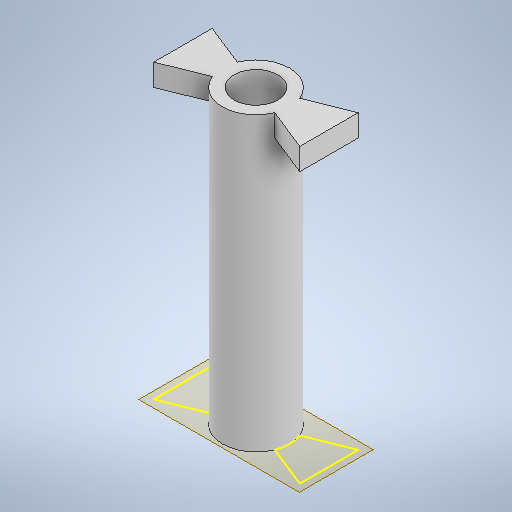
# Autodesk Inventor part: PruebaBuje
Saved by Autodesk Inventor 2025.2 (Build 292293000, 293)
## iProperties
Created: 2025-04-03
Part Number: PruebaBuje
Material: Genérico
Document SubType Name: Modeling
Designer: braug
Density: 1 g/cm^3
Appearance: Valor por defecto
Author: braug
## iProperties of the stored document PruebaBuje_3DPrint.ipt
Created: 2025-04-03
Part Number: PruebaBuje_3DPrint
Material: Genérico
Document SubType Name: Modeling
Designer: braug
Density: 1 g/cm^3
Appearance: Valor por defecto
Author: braug
Autodesk Inventor part; units mm, degrees
ref_plane "YZ Plane" through (0, 0, 0) normal (1, 0, 0) x (0, 1, 0)
ref_plane "XY Plane" through (0, 0, 0) normal (0, 0, 1) x (1, 0, 0)
sketch "Boceto1" plane through (0, 0, 0) normal (0, 1, 0) x (-1, 0, 0)
  circle A0 centre (0, 0) radius 1.5
  circle A1 centre (0, 0) radius 2.3
  dimension "d0" = 3
  dimension "d1" = 4.6
  constraints: 2 centre point, 2 coincident
  measures "d0" diameter of A0
  measures "d1" diameter of A1
extrude "Extrusión1" add sketch "Boceto1" along normal blind 20
sketch "Boceto2" plane through (0, 20, 0) normal (0, 1, 0) x (1, 0, 0)
  line L0 (5, 2) -> (5, -2)
  line L1 (-5, -2) -> (-5, 2)
  circle A0 centre (0, 0) radius 1.5 projected
  line L2 (-5, 2) -> (5, -2) construction
  line L3 (5, 2) -> (-5, -2) construction
  circle A1 centre (0, 0) radius 2.3 projected
  line L4 (-2.1355, 0.8542) -> (-5, 2)
  line L5 (-2.1355, -0.8542) -> (-5, -2)
  line L6 (2.1355, 0.8542) -> (5, 2)
  line L7 (5, -2) -> (2.1355, -0.8542)
  arc A2 (-2.1355, 0.8542) -> (-2.1355, -0.8542) centre (0, 0) ccw
  arc A3 (2.1355, -0.8542) -> (1.6097, 1.6429) centre (0, 0) ccw
  dimension "d5" = 4
  dimension "d8" = 10
  constraints: 16 end point, 8 point on circle, 4 point on line, 2 centre point, 2 collinear, 2 midpoint, 1 coincident, 1 parallel
  measures "d5" distance of L0.start L0.end
  measures "d8" distance between parallel lines of L1 L0
extrude "Extrusión2" add sketch "Boceto2" against normal blind 1.5 contours L0 L7 A1 L6 | L5 L1 L4 A1
sketch "Boceto3" plane through (0, 0, 0) normal (0, -1, 0) x (1, 0, 0)
  line L0 (-2.1355, 0.8542) -> (-5, 2) projected
  line L1 (-5, 2) -> (-5, -2) projected
  line L2 (-2.1355, 0.8542) -> (-5, 2) projected
  line L3 (-5, 2) -> (-5, -2) projected
  line L4 (-5, -2) -> (-2.1355, -0.8542) projected
  arc A0 (-2.1355, 0.8542) -> (-2.1355, -0.8542) centre (0, 0) ccw projected
  line L5 (2.1355, -0.8542) -> (5, -2) projected
  line L6 (5, -2) -> (5, 2) projected
  line L7 (5, 2) -> (2.1355, 0.8542) projected
  arc A1 (2.1355, -0.8542) -> (2.1355, 0.8542) centre (0, 0) ccw projected
